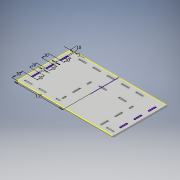
# Autodesk Inventor part: base_v2
Saved by Autodesk Inventor 2017.2 (Build 212233000, 233)
## iProperties
Created: 2017-06-08
Part Number: base_v2
Material: Generic
Document SubType Name: Modeling
Designer: SandeepSH
Density: 1 g/cm^3
Appearance: Default
Author: SandeepSH
Autodesk Inventor part; units mm, degrees
ref_plane "YZ Plane" through (0, 0, 0) normal (1, 0, 0) x (0, 1, 0)
ref_plane "XZ Plane" through (0, 0, 0) normal (0, 1, 0) x (-1, 0, 0)
ref_plane "XY Plane" through (0, 0, 0) normal (0, 0, 1) x (1, 0, 0)
sketch "Sketch1" plane through (0, 0, 0) normal (0, 1, 0) x (-1, 0, 0)
  line L0 (0, 0) -> (-270, 0)
  line L1 (-270, 0) -> (-270, -150)
  line L2 (-270, -150) -> (0, -150)
  line L3 (0, -150) -> (0, 0)
  dimension "d0" = 270
  dimension "d1" = 150
  constraints: 8 end point, 2 parallel, 1 horizontal, 1 perpendicular
  measures "d0" distance of L2.end L1.end
  measures "d1" distance of L1.end L0.end
extrude "Extrusion1" add sketch "Sketch1" along normal blind 3
fillet "Fillet1" radius 2 4 edges at (0, 1.5, 0) (270, 1.5, 0) (0, 1.5, -150) (270, 1.5, -150) curvature continuous yes
sketch "Sketch2" plane through (0, 3, 0) normal (0, 1, 0) x (1, 0, 0)
  point P0 (0, 0)
sketch "Sketch3" plane through (0, 3, 0) normal (0, 1, 0) x (1, 0, 0)
  line L0 (35, 140) -> (55, 140)
  line L1 (55, 140) -> (55, 137)
  line L2 (55, 137) -> (35, 137)
  line L3 (35, 137) -> (35, 140)
  line L4 (268, 150) -> (2, 150) projected
  line L5 (0, 148) -> (0, 2) projected
  line L6 (75, 140) -> (95, 140)
  line L7 (95, 140) -> (95, 137)
  line L8 (95, 137) -> (75, 137)
  line L9 (75, 137) -> (75, 140)
  line L10 (115, 140) -> (135, 140)
  line L11 (135, 140) -> (135, 137)
  line L12 (135, 137) -> (115, 137)
  line L13 (115, 137) -> (115, 140)
  line L14 (155, 137) -> (175, 137)
  line L15 (175, 137) -> (175, 140)
  line L16 (175, 140) -> (155, 140)
  line L17 (155, 140) -> (155, 137)
  line L18 (195, 140) -> (215, 140)
  line L19 (215, 140) -> (215, 137)
  line L20 (215, 137) -> (195, 137)
  line L21 (195, 137) -> (195, 140)
  point P0 (0, 0)
  dimension "d5" = 20
  dimension "d6" = 3
  dimension "d7" = 10
  dimension "d8" = 35
  dimension "d9" = 20
  dimension "d10" = 3
  dimension "d11" = 20
  dimension "d12" = 20
  dimension "d13" = 20
  dimension "d14" = 3
  dimension "d15" = 20
  dimension "d16" = 20
  dimension "d17" = 20
  dimension "d18" = 20
  dimension "d19" = 3
  dimension "d20" = 3
  constraints: 40 end point, 10 parallel, 5 horizontal, 5 perpendicular, 4 collinear
  measures "d5" distance of L1.end L2.end
  measures "d6" distance of L0.end L1.end
  measures "d7" distance between parallel lines of L4 L0
  measures "d8" distance between parallel lines of L3 L5
  measures "d9" distance of L7.end L8.end
  measures "d10" distance between parallel lines of L6 L8
  measures "d11" distance between parallel lines of L1 L9
  measures "d12" distance of L11.end L12.end
  measures "d13" distance between parallel lines of L7 L13
  measures "d14" distance between parallel lines of L10 L12
  measures "d15" distance of L16.end L15.end
  measures "d16" distance between parallel lines of L17 L11
  measures "d17" distance of L19.end L20.end
  measures "d18" distance between parallel lines of L21 L15
  measures "d19" distance between parallel lines of L20 L18
  measures "d20" distance between parallel lines of L14 L16
extrude "Extrusion2" cut sketch "Sketch3" against normal through all
sketch "Sketch4" plane through (0, 3, 0) normal (0, 1, 0) x (1, 0, 0)
  line L0 (10, 30) -> (13, 30)
  line L1 (13, 30) -> (13, 50)
  line L2 (13, 50) -> (10, 50)
  line L3 (10, 50) -> (10, 30)
  line L4 (2, 0) -> (268, 0) projected
  line L5 (10, 70) -> (13, 70)
  line L6 (13, 70) -> (13, 90)
  line L7 (13, 90) -> (10, 90)
  line L8 (10, 90) -> (10, 70)
  line L9 (10, 110) -> (13, 110)
  line L10 (13, 110) -> (13, 130)
  line L11 (13, 130) -> (10, 130)
  line L12 (10, 130) -> (10, 110)
  line L13 (0, 148) -> (0, 2) projected
  line L14 (135, 70) -> (135, 150)
  line L15 (268, 150) -> (2, 150) projected
  line L16 (260, 30) -> (257, 30)
  line L17 (257, 30) -> (257, 50)
  line L18 (257, 50) -> (260, 50)
  line L19 (260, 50) -> (260, 30)
  line L20 (260, 70) -> (257, 70)
  line L21 (257, 70) -> (257, 90)
  line L22 (257, 90) -> (260, 90)
  line L23 (260, 90) -> (260, 70)
  line L24 (260, 110) -> (257, 110)
  line L25 (257, 110) -> (257, 130)
  line L26 (257, 130) -> (260, 130)
  line L27 (260, 130) -> (260, 110)
  point P0 (0, 0)
  dimension "d23" = 3
  dimension "d24" = 20
  dimension "d25" = 30
  dimension "d26" = 3
  dimension "d27" = 20
  dimension "d28" = 20
  dimension "d29" = 20
  dimension "d30" = 20
  dimension "d31" = 135
  dimension "d72" = 10
  dimension "d73" = 3
  constraints: 50 end point, 12 symmetric about line, 6 parallel, 3 horizontal, 3 perpendicular, 2 collinear, 1 midpoint
  measures "d23" distance of L2.end L1.end
  measures "d24" distance of L1.end L0.end
  measures "d25" distance between parallel lines of L4 L0
  measures "d26" distance of L7.end L6.end
  measures "d27" distance of L6.end L5.end
  measures "d28" distance between parallel lines of L5 L2
  measures "d29" distance of L10.end L9.end
  measures "d30" distance between parallel lines of L9 L7
  measures "d31" distance from line of L13 L14.start
  measures "d72" distance between parallel lines of L13 L8
  measures "d73" distance between parallel lines of L12 L10
extrude "Extrusion3" cut sketch "Sketch4" against normal through all
sketch "Sketch5" plane through (0, 3, 0) normal (0, 1, 0) x (1, 0, 0)
  line L0 (224, 30) -> (227, 30)
  line L1 (227, 30) -> (227, 10)
  line L2 (227, 10) -> (224, 10)
  line L3 (224, 10) -> (224, 30)
  line L4 (257, 30) -> (257, 50) projected
  line L5 (2, 0) -> (268, 0) projected
  line L6 (224, 50) -> (227, 50)
  line L7 (227, 50) -> (227, 70)
  line L8 (227, 70) -> (224, 70)
  line L9 (224, 70) -> (224, 50)
  line L10 (224, 100) -> (227, 100)
  line L11 (227, 100) -> (227, 90)
  line L12 (227, 90) -> (224, 90)
  line L13 (224, 90) -> (224, 100)
  line L14 (166.5, 70) -> (166.5, 17.3538)
  line L15 (109, 50) -> (106, 50)
  line L16 (106, 50) -> (106, 70)
  line L17 (106, 70) -> (109, 70)
  line L18 (109, 70) -> (109, 50)
  line L19 (109, 100) -> (106, 100)
  line L20 (106, 100) -> (106, 90)
  line L21 (106, 90) -> (109, 90)
  line L22 (109, 90) -> (109, 100)
  line L23 (106, 20) -> (109, 20)
  line L24 (109, 20) -> (109, 30)
  line L25 (109, 30) -> (106, 30)
  line L26 (106, 30) -> (106, 20)
  point P0 (0, 0)
  dimension "d34" = 3
  dimension "d35" = 20
  dimension "d36" = 30
  dimension "d37" = 10
  dimension "d38" = 20
  dimension "d39" = 20
  dimension "d40" = 3
  dimension "d41" = 10
  dimension "d42" = 20
  dimension "d43" = 57.5
  dimension "d57" = 3
  dimension "d58" = 10
  dimension "d59" = 20
  constraints: 50 end point, 8 parallel, 8 symmetric about line, 4 horizontal, 4 perpendicular, 1 collinear, 1 vertical
  measures "d34" distance of L1.end L2.end
  measures "d35" distance of L0.end L1.end
  measures "d36" distance between parallel lines of L4 L1
  measures "d37" distance between parallel lines of L5 L2
  measures "d38" distance of L7.end L6.end
  measures "d39" distance between parallel lines of L0 L6
  measures "d40" distance of L11.end L12.end
  measures "d41" distance of L10.end L11.end
  measures "d42" distance between parallel lines of L8 L12
  measures "d43" distance between parallel lines of L9 L14
  measures "d57" distance of L25.end L24.end
  measures "d58" distance of L24.end L23.end
  measures "d59" distance between parallel lines of L5 L23
extrude "Extrusion4" cut sketch "Sketch5" against normal through all
sketch "Sketch6" plane through (0, 3, 0) normal (0, 1, 0) x (1, 0, 0)
  line L0 (260, 10) -> (240, 10)
  line L1 (240, 10) -> (240, 13)
  line L2 (240, 13) -> (260, 13)
  line L3 (260, 13) -> (260, 10)
  line L4 (2, 0) -> (268, 0) projected
  line L5 (270, 2) -> (270, 148) projected
  line L6 (10, 10) -> (30, 10)
  line L7 (30, 10) -> (30, 13)
  line L8 (30, 13) -> (10, 13)
  line L9 (10, 13) -> (10, 10)
  line L10 (0, 148) -> (0, 2) projected
  line L11 (50, 10) -> (70, 10)
  line L12 (70, 10) -> (70, 13)
  line L13 (70, 13) -> (50, 13)
  line L14 (50, 13) -> (50, 10)
  line L15 (99, 10) -> (109, 10)
  line L16 (109, 10) -> (109, 13)
  line L17 (109, 13) -> (99, 13)
  line L18 (99, 13) -> (99, 10)
  line L19 (109, 30) -> (109, 20) projected
  point P0 (0, 0)
  dimension "d46" = 20
  dimension "d47" = 3
  dimension "d48" = 10
  dimension "d49" = 10
  dimension "d50" = 20
  dimension "d51" = 3
  dimension "d52" = 10
  dimension "d53" = 10
  dimension "d54" = 20
  dimension "d55" = 3
  dimension "d56" = 20
  dimension "d60" = 10
  dimension "d61" = 3
  constraints: 32 end point, 8 parallel, 4 horizontal, 4 perpendicular, 1 collinear
  measures "d46" distance of L1.end L2.end
  measures "d47" distance of L0.end L1.end
  measures "d48" distance between parallel lines of L4 L0
  measures "d49" distance between parallel lines of L5 L3
  measures "d50" distance of L8.end L7.end
  measures "d51" distance of L7.end L6.end
  measures "d52" distance between parallel lines of L10 L9
  measures "d53" distance between parallel lines of L4 L6
  measures "d54" distance of L13.end L12.end
  measures "d55" distance of L12.end L11.end
  measures "d56" distance between parallel lines of L14 L7
  measures "d60" distance of L17.end L16.end
  measures "d61" distance of L16.end L15.end
extrude "Extrusion5" cut sketch "Sketch6" against normal through all
sketch "Sketch7" plane through (0, 3, 0) normal (0, 1, 0) x (1, 0, 0)
  line L0 (129, 100) -> (149, 100)
  line L1 (149, 100) -> (149, 103)
  line L2 (149, 103) -> (129, 103)
  line L3 (129, 103) -> (129, 100)
  line L4 (106, 100) -> (109, 100) projected
  line L5 (109, 100) -> (109, 90) projected
  line L6 (184, 100) -> (204, 100)
  line L7 (204, 100) -> (204, 103)
  line L8 (204, 103) -> (184, 103)
  line L9 (184, 103) -> (184, 100)
  line L10 (224, 90) -> (224, 100) projected
  point P0 (0, 0)
  dimension "d64" = 20
  dimension "d65" = 3
  dimension "d66" = 20
  dimension "d67" = 20
  dimension "d68" = 3
  dimension "d69" = 20
  constraints: 16 end point, 4 parallel, 2 horizontal, 2 perpendicular, 1 collinear
  measures "d64" distance of L2.end L1.end
  measures "d65" distance of L1.end L0.end
  measures "d66" distance between parallel lines of L3 L5
  measures "d67" distance of L8.end L7.end
  measures "d68" distance of L7.end L6.end
  measures "d69" distance between parallel lines of L7 L10
extrude "Extrusion6" cut sketch "Sketch7" against normal through all
equation "\"d9\" = d5"
equation "\"d10\" = d6"
equation "\"d11\" = d5"
equation "\"d12\" = d5"
equation "\"d13\" = d9"
equation "\"d14\" = d10"
equation "\"d15\" = d16"
equation "\"d16\" = d12"
equation "\"d18\" = d16"
equation "\"d19\" = d14"
equation "\"d20\" = d14"
equation "\"d38\" = d35"
equation "\"d42\" = d39"
equation "\"d56\" = d50"
equation "\"d66\" = d64"
equation "\"d69\" = d66"
body "Solid1"
